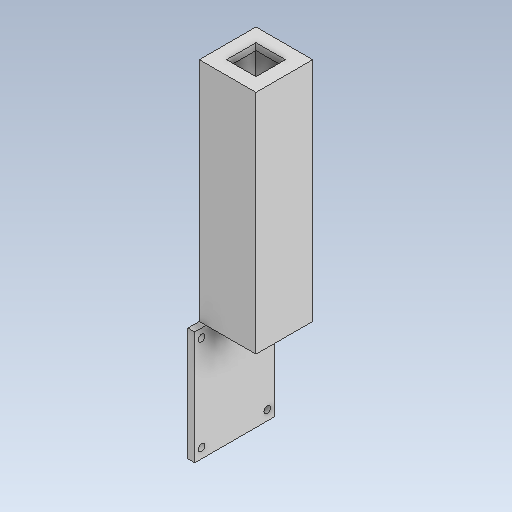
# Autodesk Inventor part: Cylinder
Saved by Autodesk Inventor 2021 (Build 250183000, 183)
## iProperties
Created: 2021-08-22
Part Number: Cylinder
Material: Generic
Document SubType Name: Modeling
Designer: techv
Density: 1 g/cm^3
Appearance: Default
Author: techv
Autodesk Inventor part; units mm, degrees
ref_plane "YZ Plane" through (0, 0, 0) normal (1, 0, 0) x (0, 1, 0)
ref_plane "XZ Plane" through (0, 0, 0) normal (0, 1, 0) x (-1, 0, 0)
ref_plane "XY Plane" through (0, 0, 0) normal (0, 0, 1) x (1, 0, 0)
sketch "Sketch1" plane through (0, 0, 0) normal (0, 1, 0) x (-1, 0, 0)
  line L0 (-12.5, 12.5) -> (12.5, 12.5)
  line L1 (12.5, 12.5) -> (12.5, -12.5)
  line L2 (12.5, -12.5) -> (-12.5, -12.5)
  line L3 (-12.5, -12.5) -> (-12.5, 12.5)
  line L4 (-12.5, 12.5) -> (12.5, -12.5) construction
  line L5 (12.5, 12.5) -> (-12.5, -12.5) construction
  line L6 (-9.5, 9.5) -> (9.5, 9.5)
  line L7 (9.5, 9.5) -> (9.5, -9.5)
  line L8 (9.5, -9.5) -> (-9.5, -9.5)
  line L9 (-9.5, -9.5) -> (-9.5, 9.5)
  line L10 (-9.5, 9.5) -> (9.5, -9.5) construction
  line L11 (9.5, 9.5) -> (-9.5, -9.5) construction
  point P0 (0, 0)
  dimension "d0" = 25
  dimension "d1" = 25
  dimension "d2" = 3
  dimension "d3" = 3
  constraints: 24 end point, 4 midpoint, 4 parallel, 2 horizontal, 2 perpendicular
  measures "d0" distance of L1.end L2.end
  measures "d1" distance of L0.end L1.end
  measures "d2" distance between parallel lines of L2 L8
  measures "d3" distance between parallel lines of L1 L7
extrude "Extrusion1" add sketch "Sketch1" along normal blind 100
sketch "Sketch2" plane through (-9.5, 0, 9.5) normal (1, 0, 0) x (0, 0, -1)
  line L0 (0, 0) -> (0, 100) projected
  line L1 (19, 0) -> (19, 100) projected
  line L2 (0, 0) -> (0, 100) projected
  line L3 (19, 0) -> (19, 100) projected
  line L4 (0, 100) -> (19, 100)
  line L5 (19, 100) -> (19, 97)
  line L6 (19, 97) -> (0, 97)
  line L7 (0, 97) -> (0, 100)
  point P0 (9.5, 0)
  point P1 (0, 97)
  point P2 (19, 97)
  dimension "d6" = 3
  constraints: 8 end point, 2 parallel, 1 horizontal, 1 perpendicular, 1 point on line
  measures "d6" distance of L4.end L5.end
extrude "Extrusion2" add sketch "Sketch2" along normal up to surface (19 mm away)
sketch "Sketch3" plane through (0, 100, 0) normal (0, 1, 0) x (1, 0, 0)
  line L0 (9.5, -9.5) -> (9.5, 9.5) projected
  line L1 (-9.5, -9.5) -> (9.5, -9.5) projected
  line L2 (-9.5, 9.5) -> (-9.5, -9.5) projected
  line L3 (9.5, 9.5) -> (-9.5, 9.5) projected
  line L4 (3.5, 3.5) -> (-3.5, 3.5)
  line L5 (-3.5, 3.5) -> (-3.5, -3.5)
  line L6 (-3.5, -3.5) -> (3.5, -3.5)
  line L7 (3.5, -3.5) -> (3.5, 3.5)
  line L8 (3.5, 3.5) -> (-3.5, -3.5) construction
  line L9 (-3.5, 3.5) -> (3.5, -3.5) construction
  line L10 (6.5, 6.5) -> (-6.5, 6.5)
  line L11 (-6.5, 6.5) -> (-6.5, -6.5)
  line L12 (-6.5, -6.5) -> (6.5, -6.5)
  line L13 (6.5, -6.5) -> (6.5, 6.5)
  line L14 (6.5, 6.5) -> (-6.5, -6.5) construction
  line L15 (-6.5, 6.5) -> (6.5, -6.5) construction
  point P0 (0, 0)
  dimension "d9" = 13
  dimension "d10" = 13
  dimension "d11" = 3
  dimension "d12" = 3
  constraints: 24 end point, 4 midpoint, 4 parallel, 2 horizontal, 2 perpendicular
  measures "d9" distance of L12.end L11.end
  measures "d10" distance of L11.end L10.end
  measures "d11" distance between parallel lines of L11 L5
  measures "d12" distance between parallel lines of L10 L4
extrude "Extrusion3" cut sketch "Sketch3" against normal blind 200 contours L7 L6 L5 L4 | L13 L12 L11 L10
sketch "Sketch4" plane through (-9.5, 0, 9.5) normal (1, 0, 0) x (0, 0, -1)
  line L0 (0, 0) -> (0, 97) projected
  line L1 (19, 0) -> (19, 97) projected
  line L2 (0, 0) -> (19, 0)
  line L3 (19, 0) -> (19, 3)
  line L4 (19, 3) -> (0, 3)
  line L5 (0, 3) -> (0, 0)
  point P0 (9.5, 0)
  dimension "d15" = 3
  constraints: 8 end point, 2 parallel, 1 horizontal, 1 perpendicular, 1 point on line
  measures "d15" distance of L3.end L2.end
extrude "Extrusion4" add sketch "Sketch4" along normal up to surface (19 mm away)
sketch "Sketch5" plane through (0, 0, 0) normal (0, -1, 0) x (1, 0, 0)
  line L0 (-6.5, 6.5) -> (6.5, 6.5) projected
  line L1 (6.5, 6.5) -> (6.5, -6.5) projected
  line L2 (6.5, -6.5) -> (-6.5, -6.5) projected
  line L3 (-6.5, -6.5) -> (-6.5, 6.5) projected
  line L4 (-9.5, -9.5) -> (9.5, -9.5) projected
  line L5 (9.5, -9.5) -> (9.5, 9.5) projected
  line L6 (9.5, 9.5) -> (-9.5, 9.5) projected
  line L7 (-9.5, 9.5) -> (-9.5, -9.5) projected
  circle A0 centre (0, 0) radius 5
  constraints: 1 centre point, 1 coincident
extrude "Extrusion5" cut sketch "Sketch5" against normal blind 200 contours A0
sketch "Sketch9" plane through (0, 0, 0) normal (0, -1, 0) x (1, 0, 0)
  circle A0 centre (0, 0) radius 9.5 projected
  point P0 (0, 0)
extrude "Extrusion9" cut sketch "Sketch9" against normal blind 10
sketch "Sketch10" plane through (0, 0, 0) normal (0, -1, 0) x (1, 0, 0)
  line L0 (12.5, -12.5) -> (-12.5, -12.5) projected
  line L1 (-12.5, -12.5) -> (-12.5, 12.5) projected
  line L2 (-12.5, -12.5) -> (-12.5, 12.5) projected
  line L3 (-12.5, 12.5) -> (-9.5, 12.5)
  line L4 (-9.5, 12.5) -> (-9.5, -12.5)
  line L5 (-9.5, -12.5) -> (-12.5, -12.5)
  line L6 (-12.5, -12.5) -> (-12.5, 12.5)
  line L7 (-6.024, 15.0194) -> (-8.024, 15.0194) projected
  line L8 (-8.024, -14.9806) -> (-6.024, -14.9806) projected
  line L9 (-12.5, 12.5) -> (12.5, 12.5) projected
  line L10 (-12.5, 12.5) -> (-9.5, 12.5)
  line L11 (-9.5, 12.5) -> (-9.5, 17.5)
  line L12 (-9.5, 17.5) -> (-12.5, 17.5)
  line L13 (-12.5, 17.5) -> (-12.5, 12.5)
  line L14 (12.5, -12.5) -> (-12.5, -12.5) projected
  line L15 (-12.5, -12.5) -> (-9.5, -12.5)
  line L16 (-9.5, -12.5) -> (-9.5, -17.5)
  line L17 (-9.5, -17.5) -> (-12.5, -17.5)
  line L18 (-12.5, -17.5) -> (-12.5, -12.5)
  point P0 (0, 0)
  point P1 (-12.5, 0)
  dimension "d53" = 3
  dimension "d54" = 25
  dimension "d55" = 5
  dimension "d56" = 5
  constraints: 24 end point, 6 parallel, 3 horizontal, 3 perpendicular, 1 midpoint, 1 point on line
  measures "d53" distance of L4.end L5.end
  measures "d54" distance of L3.end L4.end
  measures "d55" distance of L11.end L10.end
  measures "d56" distance of L15.end L16.end
extrude "Extrusion10" add sketch "Sketch10" along normal blind 50
sketch "Sketch11" plane through (-9.5, 0, -12.5) normal (1, 0, 0) x (0, 0, -1)
  line L0 (-30, 0) -> (-30, -50) construction
  line L1 (0, 0) -> (5, 0) construction
  line L2 (-30, -50) -> (5, 0) construction
  line L3 (5, 0) -> (-29.6481, 0) construction
  line L4 (-29.6481, 0) -> (5, -50) construction
  circle A0 centre (-27, -45.7143) radius 1.5
  circle A1 centre (-27, -3.8214) radius 1.5
  circle A2 centre (2, -4.2857) radius 1.5
  circle A3 centre (2, -45.6708) radius 1.5
  line L5 (5, 0) -> (5, -50) projected
  point P0 (-12.5, 0)
  dimension "d57" = 3
  dimension "d58" = 3
  dimension "d59" = 3
  dimension "d60" = 3
  dimension "d61" = 3
  dimension "d62" = 3
  dimension "d63" = 3
  dimension "d64" = 3
  constraints: 6 end point, 4 centre point, 4 point on line, 1 collinear
  measures "d57" diameter of A0
  measures "d58" diameter of A1
  measures "d59" diameter of A2
  measures "d60" diameter of A3
  measures "d61" distance from line of L5 A3.centre
  measures "d62" distance from line of L0 A0.centre
  measures "d63" distance from line of L0 A1.centre
  measures "d64" distance from line of L5 A2.centre
extrude "Extrusion11" cut sketch "Sketch11" against normal through all
body "Solid1"
